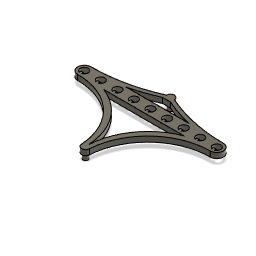
toolholder v29 (Autodesk Fusion 360 design; units mm, degrees)
Autodesk Fusion 360 part; units mm, degrees
sketch "Sketch1" plane through (0, 0, 0) normal (0, 1, 0) x (1, 0, 0)
  circle A0 centre (0, 0) radius 1.9
  circle A1 centre (0, 64) radius 1.9
  circle A2 centre (0, 0) radius 3
  circle A3 centre (0, 64) radius 3
  line L0 (0, 64) -> (0, 0)
  line L1 (0, 64) -> (0, 49)
  circle A4 centre (-50, 49) radius 5
  circle A5 centre (50, 49) radius 5
  line L2 (-50, 54) -> (50, 54)
  line L3 (-50, 44) -> (50, 44)
  circle A6 centre (0, 49) radius 5
  circle A7 centre (-25, 49) radius 5
  circle A8 centre (25, 49) radius 5
  circle A9 centre (-37.5, 49) radius 5
  circle A10 centre (-12.5, 49) radius 5
  circle A11 centre (12.5, 49) radius 5
  circle A12 centre (37.5, 49) radius 5
  line L4 (0, 64) -> (0, 61)
  line L5 (0, 61) -> (-3, 61)
  line L6 (-3, 61) -> (-3, 64)
  line L7 (0, 61) -> (3, 61)
  line L8 (3, 61) -> (3, 64)
  line L9 (0, 0) -> (-3, 0)
  line L10 (-3, 0) -> (-3, 0.173)
  line L11 (-3, 0) -> (-3, 3)
  line L12 (-3, 3) -> (0, 3)
  line L13 (0, 3) -> (3, 3)
  line L14 (3, 3) -> (3, 0)
  line L15 (-50, 44) -> (-50, 47)
  line L16 (-50, 54) -> (-50, 51)
  line L17 (50, 54) -> (50, 51)
  line L18 (50, 44) -> (50, 47)
  arc A13 (-50, 54) -> (-3, 64) centre (-50, 169.45) ccw
  arc A14 (-50, 51) -> (-3, 61) centre (-49.4067, 163.6615) ccw
  arc A15 (3, 64) -> (50, 54) centre (50, 169.45) ccw
  arc A16 (3, 61) -> (50, 51) centre (49.8725, 165.8506) ccw
  arc A17 (50, 44) -> (3, 0) centre (50, -3.1023) ccw
  arc A18 (-3, 0) -> (-50, 44) centre (-50, -3.1023) ccw
  arc A19 (0, 0) -> (-50, 47) centre (-47.09, 0) ccw
  arc A20 (50, 47) -> (0, 0) centre (47.09, 0) ccw
  dimension "d1" = 64
  dimension "d2" = 3.8
  dimension "d3" = 3.8
  dimension "d4" = 6
  dimension "d104" = 15
  dimension "d105" = 50
  dimension "d113" = 3
  dimension "d114" = 3
  dimension "d115" = 3
  dimension "d116" = 3
  dimension "d117" = 3
  dimension "d118" = 3
  dimension "d119" = 3
  dimension "d120" = 3
  dimension "d121" = 3
  constraint coincident A0.centre A2.centre
  constraint concentric A1 A3
  constraint coincident A1.centre A3.centre
  constraint vertical L0
  constraint parallel L0 L1
  constraint coincident A4 L2.start
  constraint coincident A5 L2.end
  constraint tangent A5 L2
  constraint coincident A4 L3.start
  constraint coincident A5 L3.end
  constraint tangent A5 L3
  constraint coincident L1.end A6.centre
  constraint tangent L2 A6
  constraint tangent L2 A7
  constraint tangent L2 A8
  constraint tangent L2 A9
  constraint tangent L3 A10
  constraint tangent L3 A11
  constraint tangent L3 A12
  constraint parallel L0 L4
  constraint perpendicular L1 L5
  constraint coincident A3 L6.end
  constraint tangent A3 L6
  constraint perpendicular L5 L6
  constraint perpendicular L1 L7
  constraint coincident A3 L8.end
  constraint tangent A3 L8
  constraint coincident A2 L9.end
  constraint perpendicular L0 L9
  constraint tangent A2 L10
  constraint perpendicular L9 L11
  constraint coincident L0 L12.end
  constraint coincident A2 L12.end
  constraint perpendicular L0 L13
  constraint coincident A2 L14.end
  constraint tangent A2 L14
  constraint perpendicular L3 L15
  constraint perpendicular L2 L16
  constraint perpendicular L2 L17
  constraint perpendicular L3 L18
  constraint tangent L2 A13
  constraint tangent L2 A15
  constraint tangent L3 A17
  constraint tangent L3 A18
  constraint tangent L0 A19
  constraint tangent L0 A20
  measures "d1" distance of A0.centre A1.centre
  measures "d2" diameter of A0
  measures "d3" diameter of A1
  measures "d4" diameter of A2
  measures "d104" distance of A1.centre L1.end
  measures "d105" distance of L1.end A4.centre
  measures "d113" distance of A1.centre L4.end
  measures "d114" distance of L4.end L5.end
  measures "d115" distance of L4.end L7.end
  measures "d116" distance of L9.end L11.end
  measures "d117" distance of L12.end L13.end
  measures "d118" distance of L3.start L15.end
  measures "d119" distance of L2.start L16.end
  measures "d120" distance of L2.end L17.end
  measures "d121" distance of L3.end L18.end
extrude "Extrude1" add sketch "Sketch1" along normal blind 4 contours A0 L9 A20 | A0 A2 L9 A20 | A0 L0 A20 | A0 A2 L0 L13 A20 | A0 A2 L9 A19 | A0 L9 A19 | A0 L0 A19 | A0 A2 L0 L12 A19 | A2 L13 L14 | L3 L13 L14 A17 A20 | A2 L10 L11 L12 | L3 L10 L11 L12 A18 A19 | L3 A12 A20 | L3 A8 A12 A16 A20 | A4 L15 A19 | A4 L3 A9 A19 | A4 L15 L16 A14 A19 | L0 L1 A6 | L2 L3 A6 A11 | L2 L3 A6 A10 | L0 L1 A6 | A5 L17 L18 A16 A20 | A5 L3 A12 A20 | A5 L18 A20 | L2 L3 A8 A11 A16 | A8 A16 | A12 A20 | A12 A16 A20 | L3 A7 A9 A14 A19 | L3 A9 A19 | A4 L2 A9 A14 | L2 L6 A13 A14 | A4 L16 A14 | A4 A9 A14 A19 | A9 A19 | L2 L3 A7 A10 A14 | A10 | A11 | A5 A12 A16 A20 | L2 A8 A16 | A8 A16 | L2 A8 A12 A16 | A12 A16 | A7 A14 | A9 A14 A19 | L2 A7 A9 A14 | A9 A14 | A3 | A3 L5 L6 | A3 L7 L8 | A5 L17 A16 | A5 L2 A12 A16 | L2 L8 A15 A16 | A7 A14 | L2 A7 A14 | A1
sketch "Sketch2" plane through (0, 0, 0) normal (0, -1, 0) x (1, 0, 0)
  arc A0 (-0.0956, -2.9985) -> (0, -3) centre (0, 0) ccw
  circle A1 centre (0, -64) radius 1.9
  circle A2 centre (0, 0) radius 1.9
  line L0 (0, -3) -> (0.0957, -3)
  line L1 (3, -61) -> (-3, -61)
  arc A3 (-3, -61) -> (-23.5741, -54) centre (-49.4067, -163.6615) ccw
  line L2 (-23.5741, -54) -> (23.7934, -54)
  arc A4 (23.7934, -54) -> (3, -61) centre (49.8725, -165.8506) ccw
  arc A5 (0.0957, -3) -> (30.313, -44) centre (47.09, 0) ccw
  line L3 (30.313, -44) -> (-30.313, -44)
  arc A6 (-30.313, -44) -> (-0.0956, -2.9985) centre (-47.09, 0) ccw
  arc A7 (50, -54) -> (50, -44) centre (50, -49) ccw
  arc A8 (3, 0) -> (50, -44) centre (50, 3.1023) ccw
  arc A9 (3, 0) -> (-3, 0) centre (0, 0) ccw
  arc A10 (-50, -44) -> (-3, 0) centre (-50, 3.1023) ccw
  arc A11 (-50, -44) -> (-50, -54) centre (-50, -49) ccw
  arc A12 (-3, -64) -> (-50, -54) centre (-50, -169.45) ccw
  arc A13 (-3, -64) -> (3, -64) centre (0, -64) ccw
  arc A14 (50, -54) -> (3, -64) centre (50, -169.45) ccw
  point P0 (-42.7508, -144.2813)
  dimension "d37" = 3.8
  dimension "d38" = 3.8
  measures "d37" diameter of A1
  measures "d38" diameter of A2
extrude "Extrude2" add sketch "Sketch2" along normal blind 4 contours A1 | A2
sketch "Sketch5" plane through (0, 4, 0) normal (0, 1, 0) x (-1, 0, 0)
  arc A0 (0, -3) -> (0.0956, -2.9985) centre (0, 0) ccw
  line L0 (-0.0957, -3) -> (0, -3)
  line L1 (3, -61) -> (-3, -61)
  arc A1 (-3, -61) -> (-23.7934, -54) centre (-49.8725, -165.8506) ccw
  arc A2 (23.5741, -54) -> (3, -61) centre (49.4067, -163.6615) ccw
  arc A3 (0.0956, -2.9985) -> (30.313, -44) centre (47.09, 0) ccw
  line L2 (30.313, -44) -> (-30.313, -44)
  arc A4 (-30.313, -44) -> (-0.0957, -3) centre (-47.09, 0) ccw
  arc A5 (-50, -44) -> (-50, -54) centre (-50, -49) ccw
  arc A6 (-3, -64) -> (-50, -54) centre (-50, -169.45) ccw
  arc A7 (-3, -64) -> (3, -64) centre (0, -64) ccw
  arc A8 (50, -54) -> (3, -64) centre (50, -169.45) ccw
  arc A9 (50, -54) -> (50, -44) centre (50, -49) ccw
  arc A10 (3, 0) -> (50, -44) centre (50, 3.1023) ccw
  arc A11 (3, 0) -> (-3, 0) centre (0, 0) ccw
  arc A12 (-50, -44) -> (-3, 0) centre (-50, 3.1023) ccw
  circle A13 centre (50, -49) radius 3
  circle A14 centre (-50, -49) radius 3
  line L3 (0, -44) -> (0, -54)
  circle A15 centre (0, -49) radius 3
  line L4 (0, -49) -> (25, -49)
  circle A16 centre (25, -49) radius 3
  circle A17 centre (12.5, -49) radius 3
  line L5 (25, -49) -> (50, -49)
  line L6 (0, -49) -> (-25, -49)
  line L7 (-25, -49) -> (-50, -49)
  circle A18 centre (37.5, -49) radius 3
  circle A19 centre (-12.5, -49) radius 3
  circle A20 centre (-25, -49) radius 3
  circle A21 centre (-37.5, -49) radius 3
  line L8 (50, -49) -> (50, -46)
  line L9 (50, -47.5) -> (51, -47.5)
  line L10 (50, -47.5) -> (49, -47.5)
  line L11 (49, -47.5) -> (49, -46.1716)
  line L12 (51, -47.5) -> (51, -46.1716)
  line L13 (37.5, -47.5) -> (36.5, -47.5)
  line L14 (37.5, -47.5) -> (38.5, -47.5)
  line L15 (38.5, -47.5) -> (38.5, -46.1716)
  line L16 (36.5, -47.5) -> (36.5, -46.1716)
  line L17 (25, -47.5) -> (24, -47.5)
  line L18 (25, -47.5) -> (26, -47.5)
  line L19 (26, -47.5) -> (26, -46.1716)
  line L20 (24, -47.5) -> (24, -46.1716)
  line L21 (12.5, -47.5) -> (13.5, -47.5)
  line L22 (12.5, -47.5) -> (11.5, -47.5)
  line L23 (11.5, -47.5) -> (11.5, -46.1716)
  line L24 (13.5, -47.5) -> (13.5, -46.1716)
  line L25 (0, -47.4828) -> (1, -47.4828)
  line L26 (0, -47.4828) -> (-1, -47.4828)
  line L27 (-1, -47.4828) -> (-1, -46.1716)
  line L28 (1, -47.4828) -> (1, -46.1716)
  line L29 (-12.5, -47.4828) -> (-11.5, -47.4828)
  line L30 (-12.5, -47.4828) -> (-13.5, -47.4828)
  line L31 (-13.5, -47.4828) -> (-13.5, -46.1716)
  line L32 (-11.5, -47.4828) -> (-11.5, -46.1716)
  line L33 (-25, -47.4828) -> (-24, -47.4828)
  line L34 (-25, -47.4828) -> (-26, -47.4828)
  line L35 (-26, -47.4828) -> (-26, -46.1716)
  line L36 (-24, -47.4828) -> (-24, -46.1716)
  line L37 (-37.5, -47.4828) -> (-36.5, -47.4828)
  line L38 (-37.5, -47.4828) -> (-38.5, -47.4828)
  line L39 (-38.5, -47.4828) -> (-38.5, -46.1716)
  line L40 (-36.5, -47.4828) -> (-36.5, -46.1716)
  line L41 (-50, -47.4828) -> (-49, -47.4828)
  line L42 (-50, -47.4828) -> (-51, -47.4828)
  line L43 (-51, -47.4828) -> (-51, -46.1716)
  line L44 (-49, -47.4828) -> (-49, -46.1716)
  dimension "d122" = 6
  dimension "d123" = 6
  dimension "d124" = 10
  dimension "d125" = 6
  dimension "d126" = 25
  dimension "d127" = 6
  dimension "d128" = 6
  dimension "d129" = 25
  dimension "d130" = 6
  dimension "d131" = 6
  dimension "d132" = 6
  dimension "d133" = 6
  dimension "d134" = 1
  dimension "d135" = 1
  dimension "d136" = 1
  dimension "d137" = 1
  dimension "d138" = 1
  dimension "d139" = 1
  dimension "d140" = 1
  dimension "d141" = 1
  dimension "d142" = 1
  dimension "d143" = 1
  dimension "d144" = 1
  dimension "d145" = 1
  dimension "d146" = 1
  dimension "d147" = 1
  dimension "d148" = 1
  dimension "d149" = 1
  dimension "d150" = 1
  dimension "d151" = 1
  constraint concentric A9 A13
  constraint concentric A5 A14
  constraint midpoint L2 L3.start
  constraint perpendicular L2 L3
  constraint midpoint L3 A15.centre
  constraint coincident A15.centre L4.start
  constraint perpendicular L3 L4
  constraint coincident L4.end A16.centre
  constraint midpoint L4 A17.centre
  constraint coincident A9.centre A13.centre
  constraint perpendicular L3 L6
  constraint coincident A5.centre A14.centre
  constraint midpoint L5 A18.centre
  constraint midpoint L6 A19.centre
  constraint coincident L6.end L7.start
  constraint midpoint L7 A21.centre
  constraint coincident A13 L8.end
  constraint perpendicular L5 L8
  constraint midpoint L8 L9.start
  constraint perpendicular L8 L9
  constraint perpendicular L8 L10
  constraint coincident A13 L11.end
  constraint perpendicular L10 L11
  constraint coincident A13 L12.end
  constraint perpendicular L9 L12
  constraint perpendicular L12 L13
  constraint parallel L13 L14
  constraint coincident A18 L15.end
  constraint perpendicular L14 L15
  constraint coincident A18 L16.end
  constraint perpendicular L13 L16
  constraint perpendicular L16 L17
  constraint parallel L17 L18
  constraint coincident A16 L19.end
  constraint perpendicular L18 L19
  constraint coincident A16 L20.end
  constraint perpendicular L17 L20
  constraint perpendicular L20 L21
  constraint parallel L21 L22
  constraint coincident A17 L23.end
  constraint perpendicular L22 L23
  constraint coincident A17 L24.end
  constraint perpendicular L21 L24
  constraint coincident L3 L25.start
  constraint perpendicular L3 L25
  constraint perpendicular L3 L26
  constraint coincident A15 L27.end
  constraint perpendicular L26 L27
  constraint coincident A15 L28.end
  constraint perpendicular L26 L28
  constraint perpendicular L28 L29
  constraint parallel L29 L30
  constraint coincident A19 L31.end
  constraint perpendicular L30 L31
  constraint coincident A19 L32.end
  constraint perpendicular L29 L32
  constraint perpendicular L31 L33
  constraint parallel L33 L34
  constraint coincident A20 L35.end
  constraint perpendicular L34 L35
  constraint coincident A20 L36.end
  constraint perpendicular L33 L36
  constraint perpendicular L36 L37
  constraint parallel L37 L38
  constraint coincident A21 L39.end
  constraint perpendicular L38 L39
  constraint coincident A21 L40.end
  constraint perpendicular L37 L40
  constraint perpendicular L40 L41
  constraint parallel L41 L42
  constraint coincident A14 L43.end
  constraint perpendicular L42 L43
  constraint coincident A14 L44.end
  constraint perpendicular L41 L44
  measures "d122" diameter of A13
  measures "d123" diameter of A14
  measures "d124" distance of L3.start L3.end
  measures "d125" diameter of A15
  measures "d126" distance of A15.centre L4.end
  measures "d127" diameter of A16
  measures "d128" diameter of A17
  measures "d129" distance of A15.centre L6.end
  measures "d130" diameter of A18
  measures "d131" diameter of A19
  measures "d132" diameter of A20
  measures "d133" diameter of A21
  measures "d134" distance of L9.start L9.end
  measures "d135" distance of L9.start L10.end
  measures "d136" distance of L13.start L13.end
  measures "d137" distance of L13.start L14.end
  measures "d138" distance of L17.start L17.end
  measures "d139" distance of L17.start L18.end
  measures "d140" distance of L21.start L21.end
  measures "d141" distance of L21.start L22.end
  measures "d142" distance of L25.start L25.end
  measures "d143" distance of L25.start L26.end
  measures "d144" distance of L29.start L29.end
  measures "d145" distance of L29.start L30.end
  measures "d146" distance of L33.start L33.end
  measures "d147" distance of L33.start L34.end
  measures "d148" distance of L37.start L37.end
  measures "d149" distance of L37.start L38.end
  measures "d150" distance of L41.start L41.end
  measures "d151" distance of L41.start L42.end
extrude "Extrude5" cut sketch "Sketch5" against normal blind 5 contours A13 L5 L8 L9 L12 | A13 L5 L8 L10 L11 | A14 L41 L42 L43 L44 | L3 A15 L4 L25 L28 | L3 A15 L6 L26 L27 | L3 A15 L4 | L3 A15 L6 | L4 A17 L21 L22 L23 L24 | L4 A17 | L4 A16 L5 L17 L18 L19 L20 | L4 A16 L5 | L5 A18 L13 L14 L15 L16 | L5 A18 | L6 L7 A20 | L6 L7 A20 L33 L34 L35 L36 | L6 A19 | L6 A19 L29 L30 L31 L32 | L7 A21 | L7 A21 L37 L38 L39 L40 picked at (-50.9107, -48.805)
equation "d126 = 50.000 mm / 2"
equation "d129 = 50.000 mm / 2"
